Autodesk Inventor part; units mm, degrees
(part 5 of 5)
  line L1728 (-78.8326, -37.2618) -> (-79.6226, -37.2618) projected
  line L1729 (-79.6226, -37.2618) -> (-79.6226, -36.8618) projected
  line L1730 (-79.6226, -36.8618) -> (-78.8326, -36.8618) projected
  line L1731 (-78.8326, -36.8618) -> (-78.8326, -37.2618) projected
  line L1732 (-21.3876, -19.8118) -> (-21.3876, -11.7118) construction
  line L1733 (-20.2876, -18.7118) -> (-20.2876, -12.8118)
  line L1734 (-22.4876, -12.8118) -> (-22.4876, -18.7118)
  arc A0 (-22.4876, -18.7118) -> (-20.2876, -18.7118) centre (-21.3876, -18.7118) ccw
  arc A1 (-20.2876, -12.8118) -> (-22.4876, -12.8118) centre (-21.3876, -12.8118) ccw
  point P0 (0, 0)
  point P1 (-21.3876, -15.7618)
  dimension "d4" = 8.1
  dimension "d5" = 2.2
  dimension "d6" = 8.55
  dimension "d7" = 4.275
  constraints: 8 end point, 6 point on circle, 4 tangent, 2 centre point, 2 point on line, 1 midpoint, 1 parallel, 1 vertical
  measures "d4" distance of L1732.start L1732.end
  measures "d5" diameter of A1
  measures "d6" distance from line of L8.end L6
  measures "d7" distance from line of point (-21.388, -15.762) L6
extrude "Extrusion2" add sketch "Skizze6" along normal blind 7 contours L7 A0 L14 L13 L12 L1734 L22 L21 L20 L30 L29 L28 L38 L37 L36 L46 L45 L44 L54 L53 L52 L62 L61 L60 L70 L69 L68 A1 L11 L10 L9 L72 L75 L74 L1733 L64 L67 L66 L56 L59 L58 L48 L51 L50 L40 L43 L42 L32 L35 L34 L24 L27 L26 L16 L19 L18 L5 L4 | L4 L5 A0 L7 | A0 L1734 L12 L13 L14 | L18 L19 L16 L1733 A0 | L1734 L20 L21 L22 | L26 L27 L24 L1733 | L1734 L28 L29 L30 | L34 L35 L32 L1733 | L1734 L36 L37 L38 | L42 L43 L40 L1733 | L1734 L44 L45 L46 | L50 L51 L48 L1733 | L1734 L52 L53 L54 | L58 L59 L56 L1733 | L1734 L60 L61 L62 | L66 L67 L64 L1733 | L1734 A1 L68 L69 L70 | L74 L75 L72 A1 L1733 | A1 L9 L10 L11
pattern_linear "Rechteckige Anordnung1" count 4 spacing 18.7 along (0, 0, 1) count 6 spacing 18.7 along (-1, 0, 0) of "Extrusion2"
ref_plane "Arbeitsebene1" through (-22.1876, 0, 15.7618) normal (0, 0, 1) x (1, 0, 0)
